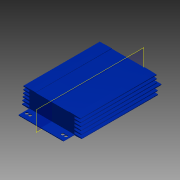
# Autodesk Inventor part: Roboteq_HDC2450
Saved by Autodesk Inventor 2012 (Build 160160000, 160)
## iProperties
Created: 2011-01-12
Part Number: Roboteq_HDC2450
Document SubType Name: Modeling
Designer: Antonella Wilby
Density: 1 g/cm^3
Material: Default
Author: Antonella Wilby
Autodesk Inventor part; units mm, degrees
ref_plane "YZ Plane" through (0, 0, 0) normal (1, 0, 0) x (0, 1, 0)
ref_plane "XY Plane" through (0, 0, 0) normal (0, 0, 1) x (1, 0, 0)
sketch "Sketch1" plane through (0, 0, 0) normal (0, 0, 1) x (1, 0, 0)
  line L0 (-124.46, 0) -> (124.46, 0) projected
  line L1 (0, -71.12) -> (0, 71.12) projected
  line L2 (-88.9, 50.8) -> (88.9, 50.8)
  line L3 (88.9, 50.8) -> (88.9, -50.8)
  line L4 (88.9, -50.8) -> (-88.9, -50.8)
  line L5 (-88.9, -50.8) -> (-88.9, 50.8)
  point P0 (0, 0)
  point P1 (-88.9, 0)
  point P2 (0, 50.8)
  dimension "d0" = 101.6
  dimension "d1" = 177.8
  constraints: 8 end point, 2 midpoint, 2 parallel, 1 horizontal, 1 horizontal alignment, 1 perpendicular, 1 vertical alignment
  measures "d0" distance of L4.end L2.start
  measures "d1" distance of L2.start L2.end
extrude "Base" add sketch "Sketch1" along normal blind 40.64
sketch "Sketch2" plane through (-88.9, -50.8, 0) normal (-1, 0, 0) x (0, 0, 1)
  line L0 (40.64, 0) -> (40.64, 101.6) projected
  line L1 (0, 0) -> (0, 101.6) projected
  line L2 (0, 0) -> (40.64, 0) projected
  line L3 (40.64, 50.8) -> (0, 50.8) construction
  line L4 (40.64, 12.7) -> (41.4337, 12.7)
  line L5 (41.4337, 12.7) -> (41.4337, 0)
  line L6 (41.4337, 0) -> (40.64, -15.4945)
  line L7 (40.64, 0) -> (40.64, -15.4945) construction
  line L8 (40.64, -15.4945) -> (0, -19.05) construction
  line L9 (40.64, -15.4945) -> (39.0525, -15.4945)
  line L10 (39.0525, -15.4945) -> (38.3401, -1.5875)
  line L11 (0, -19.05) -> (0, 0) construction
  line L12 (40.64, -1.5875) -> (0, -1.5875) construction
  line L13 (38.3401, -1.5875) -> (33.8885, -1.5875)
  line L14 (33.8885, -1.5875) -> (33.1424, -16.1504)
  line L15 (33.1424, -16.1504) -> (31.5549, -16.1504)
  line L16 (31.5549, -16.1504) -> (30.8089, -1.5875)
  line L17 (30.8089, -1.5875) -> (26.3573, -1.5875)
  line L18 (26.3573, -1.5875) -> (25.5774, -16.8123)
  line L19 (25.5774, -16.8123) -> (23.9899, -16.8123)
  line L20 (23.9899, -16.8123) -> (23.2099, -1.5875)
  line L21 (39.8463, -15.4945) -> (39.8463, -1.5875) construction
  line L22 (32.3487, -16.1504) -> (32.3487, -1.5875) construction
  line L23 (24.7836, -16.8123) -> (24.7836, -1.5875) construction
  line L24 (18.7583, -1.5875) -> (17.9442, -17.4801)
  line L25 (17.9442, -17.4801) -> (16.3567, -17.4801)
  line L26 (16.3567, -17.4801) -> (15.5425, -1.5875)
  line L27 (15.5425, -1.5875) -> (11.0909, -1.5875)
  line L28 (10.2423, -18.1539) -> (11.0909, -1.5875)
  line L29 (10.2423, -18.1539) -> (8.6548, -18.1539)
  line L30 (8.6548, -18.1539) -> (7.8061, -1.5875)
  line L31 (7.8061, -1.5875) -> (3.3545, -1.5875)
  line L32 (23.2099, -1.5875) -> (18.7583, -1.5875)
  line L33 (17.1504, -17.4801) -> (17.1504, -1.5875) construction
  line L34 (9.4485, -18.1539) -> (9.4485, -1.5875) construction
  line L35 (3.3545, -1.5875) -> (2.471, -18.8338)
  line L36 (2.471, -18.8338) -> (0.8835, -18.8338)
  line L37 (0.8835, -18.8338) -> (0, -1.5875)
  line L38 (0, -1.5875) -> (0, 0)
  line L39 (1.6772, -18.8338) -> (1.6772, -1.5875) construction
  dimension "d5" = 0.7937
  dimension "d6" = 12.7
  dimension "d7" = 5
  dimension "d11" = 1.5875
  dimension "d13" = 19.05
  dimension "d14" = 1.5875
  dimension "d16" = 5.865
  dimension "d17" = 5.865
  dimension "d18" = 5.865
  dimension "d19" = 5.865
  constraints: 72 end point, 10 parallel, 10 point on line, 9 equal length, 7 midpoint, 6 vertical, 4 collinear, 3 perpendicular, 2 horizontal, 1 coincident, 25 other
  measures "d5" distance of L4.start L4.end
  measures "d6" distance between parallel lines of L4 L2
  measures "d7" angle of L2 L8
  measures "d11" distance of L9.start L9.end
  measures "d13" distance of L8.end L1.start
  measures "d16" angle of L6 L10
  measures "d17" angle of L16 L14
  measures "d18" angle of L20 L18
  measures "d19" angle of L26 L24
extrude "Blades" add sketch "Sketch2" against normal up to surface (177.8 mm away)
mirror "Mirror1" about plane through (0, 0, 0) normal (0, 1, 0) of "Blades"
sketch "Sketch3" plane through (0, 0, 0) normal (0, 0, -1) x (-1, 0, 0)
  line L0 (88.9, -52.3875) -> (-88.9, -52.3875) projected
  line L1 (-88.9, 52.3875) -> (-114.3, 52.3875)
  line L2 (-114.3, 52.3875) -> (-114.3, -52.3875)
  line L3 (-114.3, -52.3875) -> (-88.9, -52.3875)
  line L4 (-88.9, -52.3875) -> (-88.9, 52.3875)
  line L5 (88.9, 52.3875) -> (114.3, 52.3875)
  line L6 (114.3, 52.3875) -> (114.3, -52.3875)
  line L7 (114.3, -52.3875) -> (88.9, -52.3875)
  line L8 (88.9, -52.3875) -> (88.9, 52.3875)
  point P0 (0, 0)
  dimension "d22" = 228.6
  constraints: 16 end point, 4 parallel, 3 collinear, 2 horizontal, 2 perpendicular
  measures "d22" distance between parallel lines of L6 L2
extrude "Extrusion3" add sketch "Sketch3" against normal blind 1.5875
sketch "Sketch4" plane through (0, 0, 1.5875) normal (0, 0, 1) x (1, 0, 0)
  line L0 (-114.3, 52.3875) -> (-88.9, 52.3875) projected
  line L1 (-114.3, -52.3875) -> (-114.3, 52.3875) projected
  line L2 (-101.6, 38.1) -> (-101.6, -38.1) construction
  line L3 (-101.6, -38.1) -> (-101.6, -45.72) construction
  line L4 (-101.6, 38.1) -> (-101.6, 45.72) construction
  point P0 (0, 0)
  point P1 (-101.6, 0)
  point P2 (-114.3, 0)
  point P3 (-101.6, 52.3875)
  dimension "d25" = 76.2
  dimension "d26" = 91.44
  constraints: 6 end point, 3 collinear, 3 midpoint, 2 coincident, 1 horizontal alignment, 1 parallel, 1 vertical alignment
  measures "d25" distance of L2.start L2.end
  measures "d26" distance of L3.end L4.end
hole "Mounting holes" at (-101.6, 38.1, 1.5875) at (-101.6, -38.1, 1.5875) at (-101.6, 45.72, 1.5875) at (-101.6, -45.72, 1.5875) direction (0, 0, -1) diameter 6.7564 end through all clearance for "Flat Head Machine Screw (82)" size "1/4" standard "Ansi Unified Screw Threads"
mirror "Mirror2" about plane through (0, 0, 0) normal (1, 0, 0) of "Mounting holes"
equation "\"d17\" = d16"
equation "\"d18\" = d16"
equation "\"d19\" = d16"
body "Solid1"
